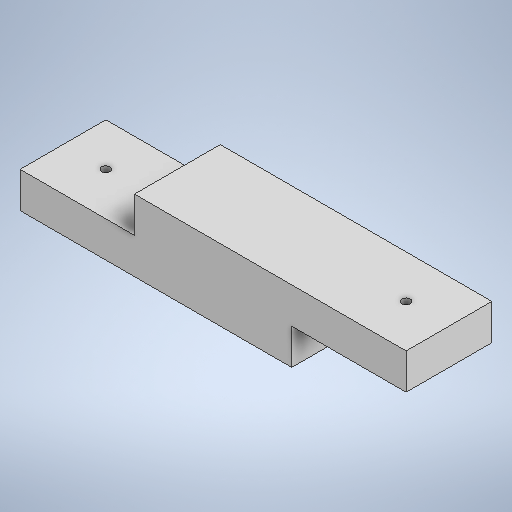
# Autodesk Inventor part: entremoteur
Saved by Autodesk Inventor 2025.2 (Build 292293000, 293)
## iProperties
Created: 2025-03-03
Part Number: entremoteur
Material: Générique
Document SubType Name: Modeling
Designer: Elisabete
Density: 1 g/cm^3
Appearance: Par défaut
Author: Elisabete
Autodesk Inventor part; units mm, degrees
ref_plane "YZ Plane" through (0, 0, 0) normal (1, 0, 0) x (0, 1, 0)
ref_plane "XZ Plane" through (0, 0, 0) normal (0, 1, 0) x (-1, 0, 0)
ref_plane "XY Plane" through (0, 0, 0) normal (0, 0, 1) x (1, 0, 0)
sketch "Esquisse1" plane through (0, 0, 0) normal (1, 0, 0) x (0, 1, 0)
  line L0 (0, 0) -> (25, 0)
  line L1 (25, 0) -> (25, -30)
  line L2 (25, -30) -> (0, -30)
  line L3 (0, -30) -> (0, 0)
  dimension "d0" = 25
  dimension "d1" = 30
  constraints: 8 end point, 2 parallel, 1 horizontal, 1 perpendicular
  measures "d0" distance of L1.end L2.end
  measures "d1" distance of L0.end L1.end
extrude "Extrusion1" add sketch "Esquisse1" along normal blind 135
sketch "Esquisse2" plane through (0, 25, 0) normal (0, 1, 0) x (1, 0, 0)
  circle A0 centre (15, 15) radius 1.5
  line L0 (0, 30) -> (135, 30) projected
  line L1 (0, 30) -> (0, 0) projected
  circle A1 centre (120, 15) radius 1.5
  line L2 (135, 30) -> (135, 0) projected
  dimension "d4" = 3
  dimension "d5" = 15
  dimension "d6" = 15
  dimension "d7" = 3
  dimension "d9" = 15
  constraints: 2 centre point
  measures "d4" diameter of A0
  measures "d5" distance from line of L0 A0.centre
  measures "d6" distance from line of L1 A0.centre
  measures "d7" diameter of A1
  measures "d9" distance from line of L2 A1.centre
extrude "Extrusion2" cut sketch "Esquisse2" against normal through all
sketch "Esquisse3" plane through (0, 0, 0) normal (0, 0, 1) x (1, 0, 0)
  line L0 (0, 25) -> (135, 25) projected
  line L1 (0, 25) -> (40, 25)
  line L2 (40, 25) -> (40, 12.5)
  line L3 (40, 12.5) -> (0, 12.5)
  line L4 (0, 12.5) -> (0, 25)
  line L5 (0, 0) -> (135, 0) projected
  line L6 (135, 0) -> (95, 0)
  line L7 (95, 0) -> (95, 12.5)
  line L8 (95, 12.5) -> (135, 12.5)
  line L9 (135, 12.5) -> (135, 0)
  dimension "d12" = 40
  dimension "d13" = 12.5
  dimension "d14" = 40
  constraints: 16 end point, 4 parallel, 2 horizontal, 2 perpendicular
  measures "d12" distance of L2.end L3.end
  measures "d13" distance of L1.end L2.end
  measures "d14" distance of L7.end L8.end
extrude "Extrusion3" cut sketch "Esquisse3" against normal through all
